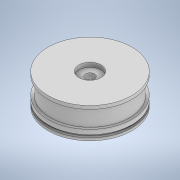
# Autodesk Inventor part: Верхняя часть поршня
Saved by Autodesk Inventor 2021 (Build 250183000, 183)
## iProperties
Created: 2020-10-24
Part Number: Верхняя часть поршня
Material: Типовые
Document SubType Name: Modeling
Designer: Тимоха
Density: 1 g/cm^3
Appearance: По умолчанию
Author: Тимоха
Autodesk Inventor part; units mm, degrees
ref_plane "YZ Plane" through (0, 0, 0) normal (1, 0, 0) x (0, 1, 0)
ref_plane "XZ Plane" through (0, 0, 0) normal (0, 1, 0) x (-1, 0, 0)
ref_plane "XY Plane" through (0, 0, 0) normal (0, 0, 1) x (1, 0, 0)
sketch "Эскиз1" plane through (0, 0, 0) normal (0, 0, 1) x (1, 0, 0)
  line L0 (49.9998, 0) -> (189, 0)
  line L1 (189, 0) -> (189, -15)
  line L2 (189, -15) -> (178, -15)
  line L3 (178, -15) -> (178, -93)
  line L4 (178, -93) -> (189, -93)
  line L5 (149, -102) -> (152.99, -56.3945)
  line L6 (137.0508, -39) -> (70.9998, -39)
  line L7 (54.9998, -55) -> (54.9998, -146)
  line L8 (24.9998, -84) -> (19.9998, -84)
  line L9 (19.9998, -84) -> (19.9998, -20)
  line L10 (19.9998, -20) -> (49.9998, -20)
  line L11 (49.9998, -20) -> (49.9998, 0)
  arc A0 (70.9998, -39) -> (54.9998, -55) centre (70.9998, -55) ccw
  arc A1 (152.99, -56.3945) -> (137.0508, -39) centre (137.0508, -55) ccw
  arc A2 (34.9998, -94) -> (24.9998, -84) centre (24.9998, -94) ccw
  line L12 (0, 0) -> (0, 25.6698)
  line L13 (189, -93) -> (189, -114)
  line L14 (189, -138) -> (169, -138)
  line L15 (169, -138) -> (169, -146)
  line L16 (169, -146) -> (149, -146)
  line L17 (189, -138) -> (189, -126)
  line L18 (189, -126) -> (178, -126)
  line L19 (178, -126) -> (178, -114)
  line L20 (178, -114) -> (189, -114)
  line L21 (189, -93) -> (189, -114)
  line L22 (149, -146) -> (149, -102)
  line L23 (54.9998, -146) -> (39.9998, -146)
  line L24 (39.9998, -146) -> (39.9998, -138)
  line L25 (39.9998, -138) -> (34.9998, -138)
  line L26 (34.9998, -138) -> (34.9998, -94)
  point P0 (154.5118, -39)
  point P1 (54.9998, -39)
  point P2 (34.9998, -84)
  dimension "d0" = 189
  dimension "d1" = 15
  dimension "d2" = 11
  dimension "d3" = 78
  dimension "d10" = 63
  dimension "d11" = 99.512
  dimension "d16" = 15
  dimension "d17" = 64
  dimension "d18" = 30
  dimension "d24" = 16
  dimension "d25" = 16
  dimension "d26" = 10
  dimension "d28" = 45
  dimension "d29" = 20
  dimension "d30" = 8
  dimension "d31" = 12
  dimension "d32" = 11
  dimension "d33" = 12
  constraints: 54 end point, 15 perpendicular, 6 point on circle, 6 point on line, 5 tangent, 4 vertical, 3 centre point, 2 horizontal, 1 collinear
  measures "d0" distance of L12.start L0.end
  measures "d1" distance of L0.end L1.end
  measures "d2" distance of L1.end L2.end
  measures "d3" distance of L2.end L3.end
  measures "d10" vertical distance of L5.start point (154.512, -39)
  measures "d11" distance of point (154.512, -39) point (55, -39)
  measures "d16" distance of point (35, -84) L8.end
  measures "d17" distance of L8.end L9.end
  measures "d18" distance of L9.end L10.end
  measures "d24" radius of A0
  measures "d25" radius of A1
  measures "d26" radius of A2
  measures "d28" distance of L14.start L4.end
  measures "d29" distance of L14.start L14.end
  measures "d30" distance of L14.end L15.end
  measures "d31" distance of L17.end L14.start
  measures "d32" distance of L17.end L18.end
  measures "d33" distance of L18.end L19.end
revolve "Вращение1" add sketch "Эскиз1" angle 360 about axis through (0, 0, 0) along (0, 1, 0)
